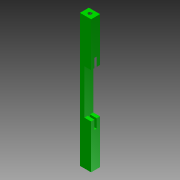
# Autodesk Inventor part: feet
Saved by Autodesk Inventor 2015 SP1 (Build 190203100, 203)
## iProperties
Created: 2011-06-09
Part Number: feet
Document SubType Name: Modeling
Designer: ijs09
Density: 1 g/cm^3
Material: Generic
Appearance: Default
Author: ijs09
Autodesk Inventor part; units mm, degrees
ref_plane "YZ Plane" through (0, 0, 0) normal (1, 0, 0) x (0, 1, 0)
ref_plane "XZ Plane" through (0, 0, 0) normal (0, 1, 0) x (-1, 0, 0)
ref_plane "XY Plane" through (0, 0, 0) normal (0, 0, 1) x (1, 0, 0)
sketch "Sketch3" plane through (0, 0, 0) normal (1, 0, 0) x (0, 1, 0)
  line L0 (-4, 59.5) -> (4, 59.5)
  line L1 (4, 59.5) -> (4, -59.5)
  line L2 (4, -59.5) -> (-4, -59.5)
  line L3 (-4, -59.5) -> (-4, 59.5)
  line L4 (-67.3512, -62.0209) -> (6.0524, -62.0209) projected
  line L5 (-86.0704, 69.3717) -> (-9.6617, 69.3717)
  line L6 (-9.4707, -54.67) -> (-85.8794, -54.67)
  point P0 (0, 0)
  dimension "d7" = 119
  dimension "d8" = 59.5
  dimension "d9" = 8
  dimension "d10" = 4
  dimension "d50" = 124.0417
  constraints: 12 end point, 3 horizontal, 2 parallel, 1 perpendicular, 4 other
  measures "d7" distance between parallel lines of L0 L2
  measures "d8" distance from line of L2 point (0, 0)
  measures "d9" distance between parallel lines of L3 L1
  measures "d10" distance from line of point (0, 0) L1
  measures "d50" distance between parallel lines of L6 L5
extrude "Extrusion1" add sketch "Sketch3" along normal blind 4
sketch "Sketch4" plane through (4, 0, 0) normal (1, 0, 0) x (0, 0, -1)
  line L0 (-59.5, 4) -> (59.5, 4) projected
  line L1 (-59.5, -4) -> (-59.5, 4) projected
  line L2 (59.5, -4) -> (-59.5, -4) projected
  line L3 (59.5, 4) -> (59.5, -4) projected
  line L4 (-59.5, 4) -> (-20, 4)
  line L5 (-20, -4) -> (-59.5, -4)
  line L6 (-59.5, -4) -> (-59.5, 4)
  line L7 (59.5, 4) -> (59.5, -4)
  line L8 (-20, 4) -> (-20, 1)
  line L9 (-20, 1) -> (-28, 1)
  line L10 (-28, 1) -> (-28, -1)
  line L11 (-28, -1) -> (-20, -1)
  line L12 (-20, -1) -> (-20, -4)
  line L13 (0, -4) -> (0, 4)
  line L14 (59.5, 4) -> (20, 4)
  line L15 (20, 1) -> (28, 1)
  line L16 (28, 1) -> (28, -1)
  line L17 (28, -1) -> (20, -1)
  line L18 (20, -1) -> (20, -4)
  line L19 (20, 4) -> (20, 1)
  line L20 (20, -4) -> (59.5, -4)
  point P0 (0, 0)
  dimension "d20" = 28
  dimension "d21" = 2
  dimension "d22" = 1
  dimension "d23" = 20
  dimension "d24" = 20
  dimension "d25" = 20
  dimension "d26" = 20
  dimension "d27" = 1
  dimension "d28" = 1
  dimension "d29" = 28
  constraints: 34 end point, 6 parallel, 3 collinear, 3 perpendicular, 3 point on line, 2 midpoint, 1 horizontal
  measures "d20" distance from line of point (0, 0) L10
  measures "d21" distance between parallel lines of L11 L9
  measures "d22" distance from line of L11 point (0, 0)
  measures "d23" distance from line of point (0, 0) L12
  measures "d24" distance from line of point (0, 0) L8
  measures "d25" distance from line of point (0, 0) L19
  measures "d26" distance from line of point (0, 0) L18
  measures "d27" distance from line of point (0, 0) L15
  measures "d28" distance from line of point (0, 0) L17
  measures "d29" distance from line of L16 point (0, 0)
extrude "Extrusion3" add sketch "Sketch4" along normal blind 6 contours L0 L8 L9 L10 L11 L12 L2 L1 | L0 L3 L2 L18 L17 L16 L15 L19
sketch "Sketch6" plane through (0, -4, 59.5) normal (0, 0, 1) x (1, 0, 0)
  line L0 (0, 8) -> (10, 8) projected
  line L1 (0, 0) -> (0, 8) projected
  point P0 (0, 4)
  point P1 (5, 4)
  dimension "d32" = 4
  dimension "d33" = 5
  measures "d32" distance from line of L0 point (5, 4)
  measures "d33" distance from line of L1 point (5, 4)
hole "Hole1" at (5, 0, 59.5) direction (0, 0, -1) diameter 3.242 depth 8.5 tip angle 118 thread size "M4x0.7" class "6H" standard "ISO Metric profile"
sketch "Sketch7" plane through (0, -4, -59.5) normal (0, 0, -1) x (-1, 0, 0)
  line L0 (0, 0) -> (-10, 0) projected
  line L1 (0, 8) -> (0, 0) projected
  point P0 (0, 4)
  point P1 (-5, 4)
  dimension "d41" = 5
  dimension "d42" = 4
  measures "d41" distance from line of L1 point (-5, 4)
  measures "d42" distance from line of point (-5, 4) L0
hole "Hole2" at (5, 0, -59.5) direction (0, 0, 1) diameter 3.242 depth 8.5 tip angle 118 thread size "M4x0.7" class "6H" standard "ISO Metric profile"
equation "\"d8\" = 0.5 * d7"
equation "\"d10\" = 0.5 * d9"
equation "\"d22\" = 0.5 * d21"
equation "\"d24\" = d23"
equation "\"d25\" = d23"
equation "\"d26\" = d23"
equation "\"d27\" = 0.5 * d21"
equation "\"d28\" = 0.5 * d21"
equation "\"d29\" = d20"
equation "\"d32\" = 0.5 * d9"
equation "\"d33\" = 0.5 * d30 + 0.5 * d11"
equation "\"d41\" = 0.5 * d30 + 0.5 * d11"
equation "\"d42\" = 0.5 * d9"
equation "\"d30\" = 6"
equation "\"d11\" = 4"
body "Solid1"
